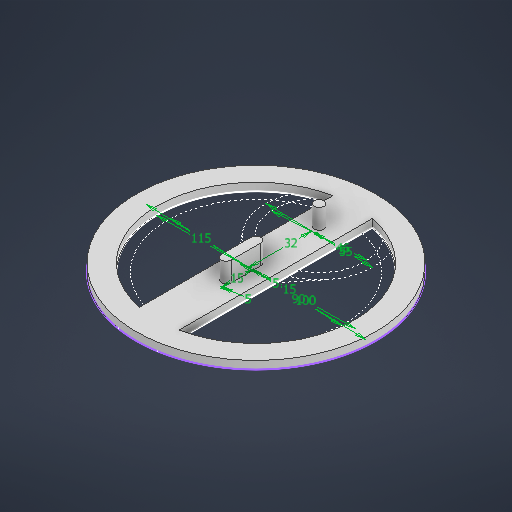
# Autodesk Inventor part: Gear Holder 2
Saved by Autodesk Inventor 2026.2 (Build 302298000, 298)
## iProperties
Created: 2026-01-26
Part Number: Gear Holder 2
Material: Generic
Document SubType Name: Modeling
Designer: Cobble
Density: 1 g/cm^3
Appearance: Default
Author: Cobble
Autodesk Inventor part; units mm, degrees
ref_plane "YZ Plane" through (0, 0, 0) normal (1, 0, 0) x (0, 1, 0)
ref_plane "XZ Plane" through (0, 0, 0) normal (0, 1, 0) x (-1, 0, 0)
ref_plane "XY Plane" through (0, 0, 0) normal (0, 0, 1) x (1, 0, 0)
sketch "Sketch1" plane through (0, 0, 0) normal (0, 0, 1) x (1, 0, 0)
  circle A0 centre (0, 0) radius 60.5278
  arc A1 (7.0788, 15.7662) -> (7.8803, 16.1398) centre (0, 32) ccw
  circle A2 centre (0, 0) radius 60.5278
  circle A3 centre (0, 32) radius 2.5
  circle A4 centre (0, 0) radius 50
  circle A5 centre (0, 0) radius 57.5 construction
  circle A6 centre (0, 0) radius 57 construction
  circle A7 centre (0, 0) radius 7.5 construction
  circle A8 centre (0, 32) radius 23 construction
  circle A9 centre (0, 0) radius 45 construction
  circle A10 centre (0, 32) radius 27.5 construction
  line L0 (-5.8547, -4.6875) -> (-21.4672, 14.8125) construction
  line L1 (5.8547, -4.6875) -> (21.4672, 14.8125) construction
  line L2 (0, 0) -> (0, 32) construction
  line L3 (7.5, 44.3706) -> (7.5, -44.3706) construction
  line L4 (-7.5, 44.3706) -> (-7.5, -44.3706) construction
  circle A11 centre (0, 0) radius 2.5
  line L5 (0, 0) -> (0, -15) construction
  circle A12 centre (0, -15) radius 2.5
  line L6 (-2.5, 0) -> (-2.5, -15)
  line L7 (2.5, -15) -> (2.5, 0)
  circle A13 centre (0, -7.5) radius 10 construction
  line L8 (-10, -7.5) -> (-10, 59.696)
  line L9 (10, -7.5) -> (10, 59.696)
  line L10 (-10, -7.5) -> (-10, -59.696)
  line L11 (10, -7.5) -> (10, -59.696)
  point P0 (35.0374, 41.2549)
  point P1 (15.3046, 2.7982)
  point P2 (-19.4282, 41.2549)
  point P3 (0.3046, 2.7982)
  point P4 (25.4129, 52.2276)
  point P5 (-9.8037, 52.2276)
  point P6 (-10, 48.9898)
  point P7 (-10, -48.9898)
  point P8 (10, 48.9898)
  point P9 (10, -48.9898)
  dimension "d0" = 5
  dimension "d1" = 100
  dimension "d2" = 115
  dimension "d3" = 15
  dimension "d4" = 46
  dimension "d5" = 90
  dimension "d6" = 55
  dimension "d7" = 32
  dimension "d8" = 5
  dimension "d9" = 15
  dimension "d10" = 5
  constraints: 24 end point, 20 point on circle, 14 centre point, 13 coincident, 12 tangent, 5 vertical, 3 parallel, 1 concentric, 1 midpoint, 1 point on line
  measures "d0" diameter of A3
  measures "d1" diameter of A4
  measures "d2" diameter of A5
  measures "d3" diameter of A7
  measures "d4" diameter of A8
  measures "d5" diameter of A9
  measures "d6" diameter of A10
  measures "d7" distance of A1.centre A0.centre
  measures "d8" diameter of A11
  measures "d9" distance of L5.start L5.end
  measures "d10" diameter of A12
extrude "Extrusion1" add sketch "Sketch1" along normal blind 4 contours A0 L11 A4 L9 | L9 A4 L8 A0 | A0 L10 A4 L11 | L8 A4 L10 A0 | L9 L11 A4 L10 L8
extrude "Extrusion2" add sketch "Sketch1" along normal blind 14 contours A3 | A11 | L7 A12 L6 A11 | A12
body "Solid1"
